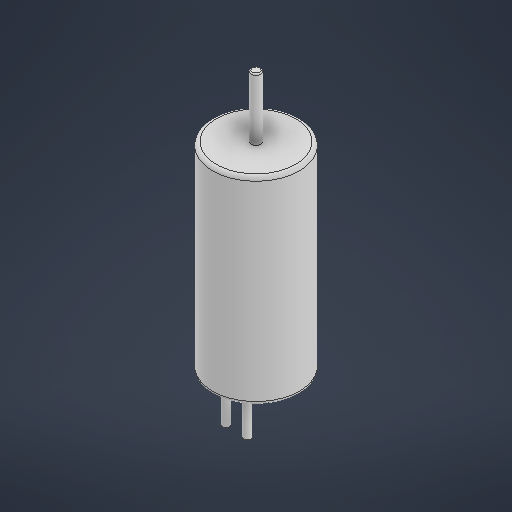
# Autodesk Inventor part: Motor
Saved by Autodesk Inventor 2027 (Build 310192000, 192)
## iProperties
Created: 2026-06-26
Part Number: Motor
Material: Genérico
Document SubType Name: Modeling
Designer: marcu
Density: 1 g/cm^3
Appearance: Padrão
Author: marcu
Autodesk Inventor part; units mm, degrees
ref_plane "YZ Plane" through (0, 0, 0) normal (1, 0, 0) x (0, 1, 0)
ref_plane "XZ Plane" through (0, 0, 0) normal (0, 1, 0) x (-1, 0, 0)
ref_plane "XY Plane" through (0, 0, 0) normal (0, 0, 1) x (1, 0, 0)
sketch "Esboço5" plane through (0, 0, 0) normal (0, 0, 1) x (1, 0, 0)
  line L0 (0, 50) -> (0, -50)
  line L1 (0, 0) -> (-3.5, 0)
  line L2 (-3.5, 0) -> (-3.5, 16)
  line L3 (-3.5, 16) -> (0, 16)
  line L4 (0, 16) -> (0, 0)
  line L5 (0, 16) -> (0, 21)
  line L6 (0, 21) -> (-0.4, 21)
  line L7 (-0.4, 21) -> (-0.4, 16)
  line L8 (-0.4, 16) -> (0, 16)
  line L9 (-2.7292, 0) -> (-2.7292, -5)
  line L10 (-0.7292, 0) -> (-0.7292, -5)
  line L11 (-0.7292, 0) -> (-0.7292, -5)
  line L12 (-0.7292, -5) -> (-1.0292, -5)
  line L13 (-1.0292, -5) -> (-1.0292, 0)
  line L14 (-1.0292, 0) -> (-0.7292, 0)
  line L15 (-2.7292, 0) -> (-2.7292, -5)
  line L16 (-2.7292, -5) -> (-2.4292, -5)
  line L17 (-2.4292, -5) -> (-2.4292, 0)
  line L18 (-2.4292, 0) -> (-2.7292, 0)
  point P0 (-1.0292, 0)
  dimension "d22" = 100
  dimension "d23" = 3.5
  dimension "d24" = 16
  dimension "d25" = 5
  dimension "d26" = 0.4
  dimension "d37" = 5
  dimension "d38" = 5
  dimension "d39" = 2
  dimension "d40" = 1.4584
  dimension "d41" = 0
  dimension "d42" = 21
  dimension "d43" = 0.8
  dimension "d44" = 5
  dimension "d45" = 5
  dimension "d46" = 0.3
  dimension "d47" = 5
  dimension "d48" = 0.3
  constraints: 38 end point, 9 parallel, 5 perpendicular, 3 point on line, 2 collinear, 2 vertical, 1 midpoint
  measures "d22" distance of L0.start L0.end
  measures "d23" distance of L1.start L1.end
  measures "d24" distance of L1.end L2.end
  measures "d25" distance of L3.end L5.end
  measures "d26" distance of L6.end L5.end
  measures "d37" distance of L9.start L9.end
  measures "d38" distance of L10.start L10.end
  measures "d39" distance between parallel lines of L10 L9
  measures "d40" diameter of L10 L0
  measures "d41" distance from line of point (0, 0) L0
  measures "d42" distance from line of point (0, 0) L6
  measures "d43" diameter of point (-0.4, 16) L0
  measures "d44" distance from line of point (-0.4, 16) L6
  measures "d45" distance of L10.start L10.end
  measures "d46" distance of L10.end L12.end
  measures "d47" distance of L9.start L9.end
  measures "d48" distance of L16.end L9.end
revolve "Revolução6" add sketch "Esboço5" angle 360 mid plane about axis through (0, 50, 0) along (0, -1, 0) contours L0 L3 L7 L6 | L0 L1 L2 L3
revolve "Revolução7" add sketch "Esboço5" angle 360 mid plane about axis through (-0.7292, 0, 0) along (0, -1, 0) contours L10 L12 L13 L1
revolve "Revolução8" add sketch "Esboço5" angle 360 mid plane about axis through (-2.4292, -5, 0) along (0, 1, 0) contours L17 L16 L9 L1
fillet "Arredondamento4" radius 0.1 1 edges at (-0.4, 21, 0)
fillet "Arredondamento5" radius 0.3 2 edges at (-3.5, 16, 0) (-3.5, 0, 0)
